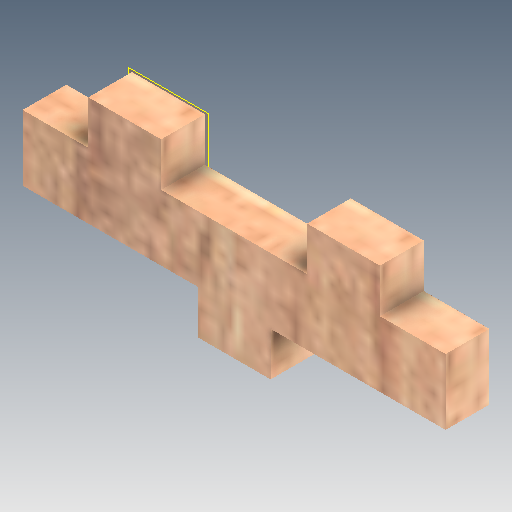
# Autodesk Inventor part: joystick buiskant
Saved by Autodesk Inventor 2020.3 (Build 243373000, 373)
## iProperties
Created: 2020-12-09
Part Number: joystick buiskant
Material: Wood (Birch)
Document SubType Name: Sheet Metal
Designer: Svend
Density: 0.55 g/cm^3
Sheet Metal Rule: Default_mm
Appearance: Birch - Natural Polished
Author: Svend
Autodesk Inventor part; units mm, degrees
ref_plane "YZ Plane" through (0, 0, 0) normal (1, 0, 0) x (0, 1, 0)
ref_plane "XZ Plane" through (0, 0, 0) normal (0, 1, 0) x (-1, 0, 0)
ref_plane "XY Plane" through (0, 0, 0) normal (0, 0, 1) x (1, 0, 0)
ref_plane "Work Plane1" through (-30, 0, 0) normal (0, 0, 1) x (1, 0, 0)
sketch "Sketch1" plane through (-30, 0, 0) normal (0, 0, 1) x (1, 0, 0)
  line L0 (0, 6) -> (10, 6)
  line L1 (0, 0) -> (0, 6)
  line L2 (10, 0) -> (0, 0)
  line L3 (10, 0) -> (10, 6)
  line L4 (30, 6) -> (40, 6)
  line L5 (30, 0) -> (30, 6)
  line L6 (40, 0) -> (30, 0)
  line L7 (40, 0) -> (40, 6)
  line L8 (49, 0) -> (49, -9)
  line L9 (-9, -9) -> (-9, 0)
  line L10 (-15, 0) -> (0, 0)
  line L11 (10, 0) -> (30, 0)
  line L12 (40, 0) -> (55, 0)
  line L13 (121.5157, 6) -> (-97.4843, 6)
  line L14 (-97.4843, -9) -> (121.5157, -9)
  line L15 (25, -9) -> (15, -9)
  line L16 (15, -9) -> (15, -15)
  line L17 (15, -15) -> (25, -15)
  line L18 (25, -15) -> (25, -9)
  point P0 (20, -15)
  point P1 (20, 0)
  dimension "d0" = 10
  dimension "d1" = 6
  measures "d0" distance of L17.end L16.end
  measures "d1" distance of L16.end L15.end
extrude "Plate1" add sketch "Sketch1" along normal blind 6 contours L0 L3 L2 L1 | L2 L11 L6 L12 L8 L14 L9 L10 | L4 L7 L6 L5 | L14 L18 L17 L16
equation "\"d2\" = Thickness"
equation "\"BendRadius\" = Thickness"
equation "\"BendReliefWidth\" = Thickness"
equation "\"BendReliefDepth\" = 0.5 * Thickness"
equation "\"CornerReliefSize\" = 4 * Thickness"
equation "\"MinimumRemnant\" = 2 * Thickness"
equation "\"TransitionRadius\" = BendRadius"
equation "\"JacobiRadiusSize\" = BendRadius"
equation "\"GapSize\" = Thickness"
equation "\"Thickness\" = 6"
body "Solid1"
